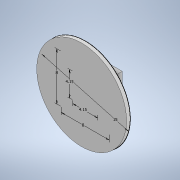
# Autodesk Inventor part: buttonBatteryConnector
Saved by Autodesk Inventor 2022 (Build 260153000, 153)
## iProperties
Created: 2022-08-03
Part Number: buttonBatteryConnector
Material: Generic
Document SubType Name: Modeling
Designer: sgioj
Density: 1 g/cm^3
Appearance: Default
Author: sgioj
Autodesk Inventor part; units mm, degrees
ref_plane "YZ Plane" through (0, 0, 0) normal (1, 0, 0) x (0, 1, 0)
ref_plane "XZ Plane" through (0, 0, 0) normal (0, 1, 0) x (-1, 0, 0)
ref_plane "XY Plane" through (0, 0, 0) normal (0, 0, 1) x (1, 0, 0)
sketch "Sketch1" plane through (0, 0, 0) normal (0, 0, 1) x (1, 0, 0)
  circle A0 centre (0, 0) radius 7.5
  line L0 (2.075, 2.075) -> (-2.075, 2.075)
  line L1 (-2.075, 2.075) -> (-2.075, -2.075)
  line L2 (-2.075, -2.075) -> (2.075, -2.075)
  line L3 (2.075, -2.075) -> (2.075, 2.075)
  line L4 (2.075, 2.075) -> (-2.075, -2.075) construction
  line L5 (-2.075, 2.075) -> (2.075, -2.075) construction
  line L6 (4, 4) -> (-4, 4)
  line L7 (-4, 4) -> (-4, -4)
  line L8 (-4, -4) -> (4, -4)
  line L9 (4, -4) -> (4, 4)
  line L10 (4, 4) -> (-4, -4) construction
  line L11 (-4, 4) -> (4, -4) construction
  dimension "d0" = 15
  dimension "d3" = 4.15
  dimension "d4" = 4.15
  dimension "d5" = 8
  dimension "d6" = 8
  constraints: 24 end point, 4 midpoint, 4 parallel, 2 horizontal, 2 perpendicular, 1 centre point, 1 coincident
  measures "d0" diameter of A0
  measures "d3" distance of L2.end L1.end
  measures "d4" distance of L1.end L0.end
  measures "d5" distance of L8.end L7.end
  measures "d6" distance of L7.end L6.end
extrude "Extrusion1" add sketch "Sketch1" along normal blind 0.6 contours A0 | L3 L2 L1 L0 | L9 L8 L7 L6
extrude "Extrusion2" add sketch "Sketch1" against normal blind 2.2 contours L9 L8 L7 L6
body "Solid1"
